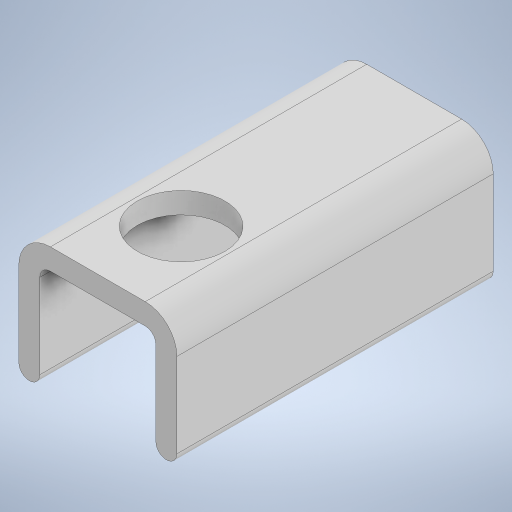
# Autodesk Inventor part: base_fotodiode
Saved by Autodesk Inventor 2024.2 (Build 282272000, 272)
## iProperties
Created: 2021-12-13
Part Number: base_fotodiode
Material: Generic
Document SubType Name: Modeling
Designer: magoo
Density: 1 g/cm^3
Appearance: Default
Description: 3D printing model
Author: magoo
Autodesk Inventor part; units mm, degrees
ref_plane "YZ Plane" through (0, 0, 0) normal (1, 0, 0) x (0, 1, 0)
ref_plane "XZ Plane" through (0, 0, 0) normal (0, 1, 0) x (-1, 0, 0)
ref_plane "XY Plane" through (0, 0, 0) normal (0, 0, 1) x (1, 0, 0)
sketch "Sketch1" plane through (0, 0, 0) normal (0, 0, 1) x (1, 0, 0)
  line L0 (5.5, -5) -> (-5.5, -5) construction
  line L1 (-5.5, -5) -> (-5.5, 5)
  line L2 (-5.5, 5) -> (5.5, 5)
  line L3 (5.5, 5) -> (5.5, -5)
  line L4 (5.5, -5) -> (-5.5, 5) construction
  line L5 (-5.5, -5) -> (5.5, 5) construction
  line L6 (-7.5, 7) -> (7.5, 7)
  line L7 (7.5, 7) -> (7.5, -5)
  line L8 (7.5, -5) -> (-7.5, -5)
  line L9 (-7.5, -5) -> (-7.5, 7)
  line L10 (0, 0) -> (0, 7) construction
  point P0 (0, 0)
  dimension "d6" = 11
  dimension "d7" = 10
  dimension "d8" = 2
  dimension "d9" = 10
  dimension "d10" = 2
  constraints: 22 end point, 4 midpoint, 4 parallel, 2 horizontal, 2 perpendicular, 1 coincident, 1 vertical
  measures "d6" distance of L1.end L2.end
  measures "d7" distance of L2.end L0.start
  measures "d8" distance between parallel lines of L6 L2
  measures "d9" distance between parallel lines of L8 L2
  measures "d10" distance between parallel lines of L7 L3
extrude "Extrusion1" add sketch "Sketch1" along normal blind 30 contours L8 L9 L6 L7 L3 L2 L1
sketch "Sketch2" plane through (-7.5, 7, 0) normal (0, 1, 0) x (1, 0, 0)
  line L0 (7.5, 0) -> (7.5, -30) construction
  line L1 (15, -30) -> (0, -30) construction
  circle A0 centre (7.5, -22.1) radius 4.15
  dimension "d14" = 7.9
  dimension "d15" = 8.3
  constraints: 2 end point, 1 centre point, 1 midpoint, 1 point on line
  measures "d14" distance from line of L1 A0.centre
  measures "d15" diameter of A0
extrude "Extrusion2" cut sketch "Sketch2" against normal up to next
sketch "Sketch3" plane through (0, 0, 0) normal (0, 0, 1) x (1, 0, 0)
  line L0 (-7.5, 7) -> (-7.5, -5) construction
  line L1 (7.5, -5) -> (7.5, 7) construction
  line L2 (5.5, -5) -> (7.5, -5) construction
  line L3 (7.5, 7) -> (-7.5, 7) construction
  line L4 (-7.5, -5) -> (-5.5, -5) construction
  line L5 (5.5, 5) -> (5.5, -5) construction
  line L6 (-5.5, -5) -> (5.5, -5) construction
  line L7 (0, -5) -> (0, 7)
  line L8 (-4.15, 7) -> (4.15, 7) construction
  line L9 (-7.5, 7) -> (-7.5, -5) construction
  line L10 (-7.5, 0) -> (7.5, 0)
  point P0 (0, 0)
  constraints: 6 end point, 3 midpoint, 2 perpendicular, 2 point on line
fillet "Fillet1" radius 1 6 edges at (-5.5, -5, 15) (-7.5, -5, 15) (5.5, -5, 15) (7.5, -5, 15) (-5.5, 5, 15) (5.5, 5, 15)
fillet "Fillet4" radius 3 2 edges at (-7.5, 7, 15) (7.5, 7, 15)
body "Solid1"
